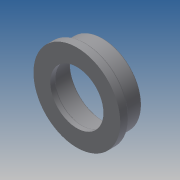
# Autodesk Inventor part: beltPulley
Saved by Autodesk Inventor 2014 (Build 180170000, 170)
## iProperties
Created: 2014-01-23
Part Number: beltPulley
Material: Generic
Document SubType Name: Modeling
Designer: Peele
Density: 1 g/cm^3
Appearance: Default
Author: Peele
Autodesk Inventor part; units mm, degrees
ref_plane "YZ Plane" through (0, 0, 0) normal (1, 0, 0) x (0, 1, 0)
ref_plane "XZ Plane" through (0, 0, 0) normal (0, 1, 0) x (-1, 0, 0)
ref_plane "XY Plane" through (0, 0, 0) normal (0, 0, 1) x (1, 0, 0)
sketch "Sketch1" plane through (0, 0, 0) normal (0, 0, 1) x (1, 0, 0)
  line L0 (0, 0) -> (0, 10.0763) construction
  line L1 (11.1, 9) -> (11.1, 2)
  line L2 (11.1, 2) -> (9.1, 2)
  line L3 (9.1, 2) -> (9.1, 0)
  line L4 (9.1, 0) -> (14.875, 0)
  line L5 (14.875, 0) -> (14.875, 3)
  line L6 (14.875, 3) -> (13.26, 3)
  line L7 (13.26, 3) -> (13.26, 9)
  line L8 (13.26, 9) -> (11.1, 9)
  dimension "d0" = 2
  dimension "d1" = 7
  dimension "d2" = 13.26
  dimension "d3" = 14.875
  dimension "d4" = 6
  dimension "d5" = 11.1
  dimension "d6" = 2
  constraints: 18 end point, 7 parallel, 1 perpendicular, 1 point on line, 1 vertical
  measures "d0" distance of L2.end L3.end
  measures "d1" distance of L1.start L1.end
  measures "d2" distance between parallel lines of L0 L7
  measures "d3" distance between parallel lines of L0 L5
  measures "d4" distance of L6.end L7.end
  measures "d5" distance between parallel lines of L0 L1
  measures "d6" distance between parallel lines of L1 L3
revolve "Revolution1" add sketch "Sketch1" angle 360 about axis through (0, 0, 0) along (0, 1, 0)
fillet "Fillet1" radius 0.5 4 edges at (-13.26, 9, 0) (-11.1, 9, 0) (-14.875, 3, 0) (-9.1, 2, 0)
body "Solid1"
